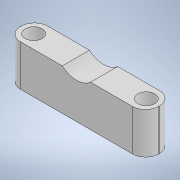
# Autodesk Inventor part: Стойка подшипника 3мм
Saved by Autodesk Inventor 2020 (Build 240168000, 168)
## iProperties
Created: 2021-05-10
Part Number: Стойка подшипника 3мм
Material: Типовые
Document SubType Name: Modeling
Designer: Антон
Density: 1 g/cm^3
Appearance: По умолчанию
Author: Антон
Autodesk Inventor part; units mm, degrees
ref_plane "YZ Plane" through (0, 0, 0) normal (1, 0, 0) x (0, 1, 0)
ref_plane "XZ Plane" through (0, 0, 0) normal (0, 1, 0) x (-1, 0, 0)
ref_plane "XY Plane" through (0, 0, 0) normal (0, 0, 1) x (1, 0, 0)
sketch "Эскиз1" plane through (0, 0, 0) normal (0, 0, 1) x (1, 0, 0)
  circle A0 centre (0, 0) radius 4.05
  line L0 (-6.05, -6.05) -> (6.05, -6.05)
  line L1 (6.05, -6.05) -> (6.05, 6.05)
  line L2 (6.05, 6.05) -> (-6.05, 6.05)
  line L3 (-6.05, 6.05) -> (-6.05, -6.05)
  line L4 (-6.05, -6.05) -> (6.05, 6.05) construction
  line L5 (6.05, -6.05) -> (-6.05, 6.05) construction
  line L6 (0, 6.05) -> (0, 4.05)
  line L7 (-6.05, 0) -> (-4.05, 0)
  line L8 (-13, -3.05) -> (0, -3.05)
  line L9 (0, -3.05) -> (0, -6.05)
  line L10 (0, -6.05) -> (-13, -6.05)
  line L11 (-13, -6.05) -> (-13, -3.05)
  line L12 (13, -3.05) -> (0, -3.05)
  line L13 (0, -6.05) -> (13, -6.05)
  line L14 (13, -6.05) -> (13, -3.05)
  point P0 (0, -4.55)
  point P1 (0, -6.05)
  point P2 (2.6646, -3.05)
  point P3 (-2.6646, -3.05)
  dimension "d0" = 8.1
  dimension "d1" = 2
  dimension "d2" = 2
  dimension "d3" = 3
  dimension "d5" = 3
  dimension "d6" = 6.95
  constraints: 30 end point, 6 midpoint, 4 parallel, 3 perpendicular, 2 horizontal, 2 point on circle, 2 symmetric about line, 1 centre point, 1 coincident, 1 vertical, 1 vertical alignment
  measures "d0" diameter of A0
  measures "d1" distance of L6.start L6.end
  measures "d2" distance of L7.start L7.end
  measures "d3" distance between parallel lines of L8 L0
  measures "d5" distance between parallel lines of L8 L10
  measures "d6" distance between parallel lines of L3 L11
extrude "Выдавливание1" add sketch "Эскиз1" along normal blind 5.1 contours L12 L1 L0 L9 A0 | L9 L0 L3 L8 A0 | L12 L14 L13 L1 | L3 L10 L11 L8
sketch "Эскиз2" plane through (-13, -3.05, 0) normal (0, 1, 0) x (1, 0, 0)
  line L0 (0, 0) -> (0, -5.1) projected
  line L1 (0, -2.55) -> (2.4, -2.55)
  point P0 (13, 0)
  dimension "d9" = 2.4
  constraints: 2 end point, 1 horizontal, 1 midpoint
  measures "d9" distance of L1.start L1.end
ref_plane "РабПлоскость1" through (0, -6.05, 0) normal (1, 0, 0) x (0, 0, -1)
hole "Отверстие1" at (-10.6, -3.05, 2.55) direction (0, -1, 0) diameter 3.2 end through all
mirror "Зеркальное отражение1" about plane through (0, -6.05, 0) normal (1, 0, 0) of "Отверстие1"
fillet "Сопряжение1" radius 2.45 4 edges at (-13, -4.55, 5.1) (-13, -4.55, 0) (13, -4.55, 5.1) (13, -4.55, 0)
sketch "Эскиз3" plane through (-10.55, -6.05, 0) normal (0, -1, 0) x (1, 0, 0)
  arc A0 (21.1, 0) -> (23.55, 2.45) centre (21.1, 2.45) ccw projected
  line L0 (0, 5.1) -> (21.1, 5.1) projected
  arc A1 (-2.45, 2.45) -> (0, 0) centre (0, 2.45) ccw projected
  line L1 (0, 0) -> (21.1, 0) projected
  circle A2 centre (-0.05, 2.55) radius 1.6 projected
  circle A3 centre (21.15, 2.55) radius 1.6 projected
  arc A4 (23.55, 2.65) -> (21.1, 5.1) centre (21.1, 2.65) ccw projected
  arc A5 (0, 5.1) -> (-2.45, 2.65) centre (0, 2.65) ccw projected
  line L2 (23.55, 2.45) -> (23.55, 2.65) projected
  line L3 (-2.45, 2.45) -> (-2.45, 2.65) projected
  point P0 (10.55, 0)
extrude "Выдавливание2" add sketch "Эскиз3" along normal blind 4.75
